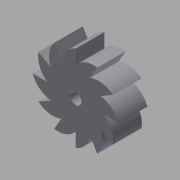
# Autodesk Inventor part: ratchet prototype
Saved by Autodesk Inventor 2013 (Build 170138000, 138)
## iProperties
Created: 2014-01-04
Part Number: ratchet prototype
Material: Generic
Document SubType Name: Modeling
Designer: kahohbein
Density: 1 g/cm^3
Author: kahohbein
Autodesk Inventor part; units mm, degrees
ref_plane "YZ Plane" through (0, 0, 0) normal (1, 0, 0) x (0, 1, 0)
ref_plane "XZ Plane" through (0, 0, 0) normal (0, 1, 0) x (-1, 0, 0)
ref_plane "XY Plane" through (0, 0, 0) normal (0, 0, 1) x (1, 0, 0)
sketch "Sketch1" plane through (0, 0, 0) normal (0, 0, 1) x (1, 0, 0)
  arc A0 (4.5113, -11.8717) -> (6.35, -10.9985) centre (0, 0) ccw
  line L0 (6.35, 10.9985) -> (9.525, 16.4978)
  line L1 (12.7, 0) -> (19.05, 0) construction
  line L2 (10.9985, 6.35) -> (16.4978, 9.525)
  line L3 (0, 0) -> (19.05, 0) construction
  line L4 (0, 12.7) -> (0, 19.05)
  line L5 (-6.35, 10.9985) -> (-9.525, 16.4978)
  line L6 (0, 0) -> (19.05, 0) construction
  line L7 (-10.9985, 6.35) -> (-16.4978, 9.525)
  line L8 (12.7, 0) -> (26.2861, 0) construction
  line L9 (0, 0) -> (19.05, 0)
  line L10 (-12.7, 0) -> (-19.05, 0)
  line L11 (6.35, -10.9985) -> (9.525, -16.4978)
  line L12 (10.9985, -6.35) -> (16.4978, -9.525)
  line L13 (0, -12.7) -> (0, -19.05)
  line L14 (-6.35, -10.9985) -> (-9.525, -16.4978)
  line L15 (-10.9985, -6.35) -> (-16.4978, -9.525)
  arc A1 (16.4978, -9.525) -> (12.7, 0) centre (6.7257, -7.9017) ccw
  arc A2 (19.05, 0) -> (10.9985, 6.35) centre (9.7755, -3.4802) ccw
  arc A3 (16.4978, 9.525) -> (6.35, 10.9985) centre (10.2059, 1.8738) ccw
  arc A4 (9.525, 16.4978) -> (0, 12.7) centre (7.9017, 6.7257) ccw
  arc A5 (0, -19.05) -> (6.35, -10.9985) centre (-3.4802, -9.7755) ccw
  arc A6 (9.525, -16.4978) -> (10.9985, -6.35) centre (1.8738, -10.2059) ccw
  arc A7 (0, 19.05) -> (-6.35, 10.9985) centre (3.4802, 9.7755) ccw
  arc A8 (-9.525, 16.4978) -> (-10.9985, 6.35) centre (-1.8738, 10.2059) ccw
  arc A9 (-9.525, -16.4978) -> (0, -12.7) centre (-7.9017, -6.7257) ccw
  arc A10 (-16.4978, -9.525) -> (-6.35, -10.9985) centre (-10.2059, -1.8738) ccw
  arc A11 (-19.05, 0) -> (-10.9985, -6.35) centre (-9.7755, 3.4802) ccw
  arc A12 (-16.4978, 9.525) -> (-12.7, 0) centre (-6.7257, 7.9017) ccw
  dimension "d0" = 25.4
  dimension "d1" = 19.05
  dimension "d2" = 60
  dimension "d3" = 19.05
  dimension "d4" = 30
  dimension "d5" = 19.05
  dimension "d6" = 120
  dimension "d7" = 150
  dimension "d8" = 9.906
  dimension "d9" = 9.906
  dimension "d10" = 9.906
  dimension "d11" = 9.906
  dimension "d18" = 9.906
  dimension "d19" = 9.906
  dimension "d20" = 9.906
  dimension "d21" = 9.906
  dimension "d22" = 9.906
  dimension "d23" = 9.906
  dimension "d24" = 9.906
  dimension "d25" = 9.906
  constraints: 32 end point, 27 point on circle, 13 centre point, 5 symmetric about line, 4 horizontal, 3 coincident, 2 collinear, 1 perpendicular, 1 point on line
  measures "d0" diameter of A0
  measures "d1" distance of L3.start L0.end
  measures "d2" angle of L1 L0
  measures "d3" distance of L3.start L2.end
  measures "d4" angle of L3 L2
  measures "d5" distance of L3.start L4.end
  measures "d6" angle of L6 L5
  measures "d7" angle of L8 L7
  measures "d8" radius of A1
  measures "d9" radius of A2
  measures "d10" radius of A3
  measures "d11" radius of A4
  measures "d18" radius of A5
  measures "d19" radius of A6
  measures "d20" radius of A7
  measures "d21" radius of A8
  measures "d22" radius of A9
  measures "d23" radius of A10
  measures "d24" radius of A11
  measures "d25" radius of A12
extrude "Extrusion1" add sketch "Sketch1" along normal blind 12.7
sketch "Sketch2" plane through (0, 0, 12.7) normal (0, 0, 1) x (1, 0, 0)
  circle A0 centre (0, 0) radius 2.54
  dimension "d28" = 5.08
  constraints: 1 centre point, 1 coincident
  measures "d28" diameter of A0
extrude "Extrusion2" cut sketch "Sketch2" against normal blind 12.7
body "Solid1"
